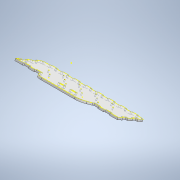
# Autodesk Inventor part: wooden_top
Saved by Autodesk Inventor 2020 (Build 240168000, 168)
## iProperties
Created: 2019-07-24
Part Number: wooden_top
Material: Generic
Document SubType Name: Modeling
Designer: erwin
Density: 1 g/cm^3
Appearance: Default
Author: erwin
Autodesk Inventor part; units mm, degrees
ref_plane "YZ Plane" through (0, 0, 0) normal (1, 0, 0) x (0, 1, 0)
ref_plane "XZ Plane" through (0, 0, 0) normal (0, 1, 0) x (-1, 0, 0)
ref_plane "XY Plane" through (0, 0, 0) normal (0, 0, 1) x (1, 0, 0)
ref_plane "Work Plane2" through (0, 481.1893, 141.342) normal (0, -0.866, 0.5) x (1, 0, 0)
sketch "Sketch2" plane through (0, 481.1893, 141.342) normal (0, -0.866, 0.5) x (1, 0, 0)
  line L0 (0, 0) -> (0, 36) projected
  line L1 (0, 0) -> (12, 0) projected
  line L2 (12, 36) -> (12, 0) projected
  line L3 (0, 36) -> (12, 36) projected
  line L4 (0, -72) -> (0, -36) projected
  line L5 (0, -72) -> (12, -72) projected
  line L6 (12, -36) -> (12, -72) projected
  line L7 (0, -36) -> (12, -36) projected
  line L8 (0, -144) -> (0, -108) projected
  line L9 (0, -144) -> (12, -144) projected
  line L10 (12, -108) -> (12, -144) projected
  line L11 (0, -108) -> (12, -108) projected
  line L12 (48, -147.6081) -> (12, -147.6081) projected
  line L13 (12, 36) -> (624, 36)
  line L14 (624, 36) -> (624, -164)
  line L15 (624, -164) -> (12, -164)
  line L16 (12, -164) -> (12, 36)
  line L17 (318, -164) -> (318, 36) construction
  line L18 (636, 0) -> (636, 36)
  line L19 (636, 0) -> (624, 0)
  line L20 (624, 36) -> (624, 0)
  line L21 (636, 36) -> (624, 36)
  line L22 (636, -72) -> (636, -36)
  line L23 (636, -72) -> (624, -72)
  line L24 (624, -36) -> (624, -72)
  line L25 (636, -36) -> (624, -36)
  line L26 (636, -144) -> (636, -108)
  line L27 (636, -144) -> (624, -144)
  line L28 (624, -108) -> (624, -144)
  line L29 (636, -108) -> (624, -108)
  line L30 (588, -147.6081) -> (624, -147.6081)
  line L31 (624, -164) -> (624, 36)
  line L32 (12, 36) -> (48, 36)
  line L33 (48, 36) -> (48, 24)
  line L34 (48, 24) -> (12, 24)
  line L35 (12, 24) -> (12, 36)
  line L36 (84, 24) -> (48, 24)
  line L37 (84, 36) -> (84, 24)
  line L38 (48, 36) -> (84, 36)
  line L39 (48, 24) -> (48, 36)
  line L40 (120, 24) -> (84, 24)
  line L41 (120, 36) -> (120, 24)
  line L42 (84, 36) -> (120, 36)
  line L43 (84, 24) -> (84, 36)
  line L44 (156, 24) -> (120, 24)
  line L45 (156, 36) -> (156, 24)
  line L46 (120, 36) -> (156, 36)
  line L47 (120, 24) -> (120, 36)
  line L48 (192, 24) -> (156, 24)
  line L49 (192, 36) -> (192, 24)
  line L50 (156, 36) -> (192, 36)
  line L51 (156, 24) -> (156, 36)
  line L52 (228, 24) -> (192, 24)
  line L53 (228, 36) -> (228, 24)
  line L54 (192, 36) -> (228, 36)
  line L55 (192, 24) -> (192, 36)
  line L56 (264, 24) -> (228, 24)
  line L57 (264, 36) -> (264, 24)
  line L58 (228, 36) -> (264, 36)
  line L59 (228, 24) -> (228, 36)
  line L60 (300, 24) -> (264, 24)
  line L61 (300, 36) -> (300, 24)
  line L62 (264, 36) -> (300, 36)
  line L63 (264, 24) -> (264, 36)
  line L64 (336, 24) -> (300, 24)
  line L65 (336, 36) -> (336, 24)
  line L66 (300, 36) -> (336, 36)
  line L67 (300, 24) -> (300, 36)
  line L68 (372, 24) -> (336, 24)
  line L69 (372, 36) -> (372, 24)
  line L70 (336, 36) -> (372, 36)
  line L71 (336, 24) -> (336, 36)
  line L72 (408, 24) -> (372, 24)
  line L73 (408, 36) -> (408, 24)
  line L74 (372, 36) -> (408, 36)
  line L75 (372, 24) -> (372, 36)
  line L76 (444, 24) -> (408, 24)
  line L77 (444, 36) -> (444, 24)
  line L78 (408, 36) -> (444, 36)
  line L79 (408, 24) -> (408, 36)
  line L80 (480, 24) -> (444, 24)
  line L81 (480, 36) -> (480, 24)
  line L82 (444, 36) -> (480, 36)
  line L83 (444, 24) -> (444, 36)
  line L84 (516, 24) -> (480, 24)
  line L85 (516, 36) -> (516, 24)
  line L86 (480, 36) -> (516, 36)
  line L87 (480, 24) -> (480, 36)
  line L88 (552, 24) -> (516, 24)
  line L89 (552, 36) -> (552, 24)
  line L90 (516, 36) -> (552, 36)
  line L91 (516, 24) -> (516, 36)
  line L92 (588, 24) -> (552, 24)
  line L93 (588, 36) -> (588, 24)
  line L94 (552, 36) -> (588, 36)
  line L95 (552, 24) -> (552, 36)
  line L96 (624, 24) -> (588, 24)
  line L97 (624, 36) -> (624, 24)
  line L98 (588, 36) -> (624, 36)
  line L99 (588, 24) -> (588, 36)
  line L100 (660, 24) -> (624, 24)
  line L101 (660, 36) -> (660, 24)
  line L102 (624, 36) -> (660, 36)
  line L103 (624, 24) -> (624, 36)
  line L104 (696, 24) -> (660, 24)
  line L105 (696, 36) -> (696, 24)
  line L106 (660, 36) -> (696, 36)
  line L107 (660, 24) -> (660, 36)
  line L108 (732, 24) -> (696, 24)
  line L109 (732, 36) -> (732, 24)
  line L110 (696, 36) -> (732, 36)
  line L111 (696, 24) -> (696, 36)
  line L112 (12, -64) -> (624, -64) construction
  line L113 (12, -164) -> (12, -128)
  line L114 (12, -164) -> (624, -164)
  line L115 (12, -164) -> (48, -164)
  line L116 (48, -164) -> (48, -152)
  line L117 (48, -152) -> (12, -152)
  line L118 (12, -152) -> (12, -164)
  line L119 (84, -152) -> (48, -152)
  line L120 (84, -164) -> (84, -152)
  line L121 (48, -164) -> (84, -164)
  line L122 (48, -152) -> (48, -164)
  line L123 (120, -152) -> (84, -152)
  line L124 (120, -164) -> (120, -152)
  line L125 (84, -164) -> (120, -164)
  line L126 (84, -152) -> (84, -164)
  line L127 (156, -152) -> (120, -152)
  line L128 (156, -164) -> (156, -152)
  line L129 (120, -164) -> (156, -164)
  line L130 (120, -152) -> (120, -164)
  line L131 (192, -152) -> (156, -152)
  line L132 (192, -164) -> (192, -152)
  line L133 (156, -164) -> (192, -164)
  line L134 (156, -152) -> (156, -164)
  line L135 (228, -152) -> (192, -152)
  line L136 (228, -164) -> (228, -152)
  line L137 (192, -164) -> (228, -164)
  line L138 (192, -152) -> (192, -164)
  line L139 (264, -152) -> (228, -152)
  line L140 (264, -164) -> (264, -152)
  line L141 (228, -164) -> (264, -164)
  line L142 (228, -152) -> (228, -164)
  line L143 (300, -152) -> (264, -152)
  line L144 (300, -164) -> (300, -152)
  line L145 (264, -164) -> (300, -164)
  line L146 (264, -152) -> (264, -164)
  line L147 (336, -152) -> (300, -152)
  line L148 (336, -164) -> (336, -152)
  line L149 (300, -164) -> (336, -164)
  line L150 (300, -152) -> (300, -164)
  line L151 (372, -152) -> (336, -152)
  line L152 (372, -164) -> (372, -152)
  line L153 (336, -164) -> (372, -164)
  line L154 (336, -152) -> (336, -164)
  line L155 (408, -152) -> (372, -152)
  line L156 (408, -164) -> (408, -152)
  line L157 (372, -164) -> (408, -164)
  line L158 (372, -152) -> (372, -164)
  line L159 (444, -152) -> (408, -152)
  line L160 (444, -164) -> (444, -152)
  line L161 (408, -164) -> (444, -164)
  line L162 (408, -152) -> (408, -164)
  line L163 (480, -152) -> (444, -152)
  line L164 (480, -164) -> (480, -152)
  line L165 (444, -164) -> (480, -164)
  line L166 (444, -152) -> (444, -164)
  line L167 (516, -152) -> (480, -152)
  line L168 (516, -164) -> (516, -152)
  line L169 (480, -164) -> (516, -164)
  line L170 (480, -152) -> (480, -164)
  line L171 (552, -152) -> (516, -152)
  line L172 (552, -164) -> (552, -152)
  line L173 (516, -164) -> (552, -164)
  line L174 (516, -152) -> (516, -164)
  line L175 (588, -152) -> (552, -152)
  line L176 (588, -164) -> (588, -152)
  line L177 (552, -164) -> (588, -164)
  line L178 (552, -152) -> (552, -164)
  line L179 (624, -152) -> (588, -152)
  line L180 (624, -164) -> (624, -152)
  line L181 (588, -164) -> (624, -164)
  line L182 (588, -152) -> (588, -164)
  line L183 (624, -152) -> (624, -164)
  circle A0 centre (318, -64) radius 2.5
  circle A1 centre (218, -64) radius 2.5
  circle A2 centre (118, -64) radius 2.5
  line L184 (624, -64) -> (12, -64) construction
  circle A3 centre (318, -64) radius 2.5
  circle A4 centre (418, -64) radius 2.5
  circle A5 centre (518, -64) radius 2.5
  circle A6 centre (168, -14) radius 2.5
  circle A7 centre (268, -14) radius 2.5
  circle A8 centre (468, -14) radius 2.5
  circle A9 centre (368, -14) radius 2.5
  line L185 (318, 36) -> (318, -164) construction
  circle A10 centre (168, -114) radius 2.5
  circle A11 centre (268, -114) radius 2.5
  circle A12 centre (468, -114) radius 2.5
  circle A13 centre (368, -114) radius 2.5
  point P0 (0, -363.0004)
  point P1 (48, 24)
  point P2 (12, 0)
  point P3 (12, -72)
  point P4 (12, -108)
  point P5 (12, -144)
  point P6 (12, -152)
  point P7 (48, -164)
  point P8 (84, -164)
  point P9 (84, -152)
  point P10 (120, -164)
  point P11 (156, -164)
  point P12 (156, -152)
  point P13 (192, -164)
  point P14 (228, -164)
  point P15 (228, -152)
  point P16 (264, -164)
  point P17 (300, -164)
  point P18 (300, -152)
  point P19 (336, -164)
  point P20 (372, -164)
  point P21 (372, -152)
  point P22 (408, -164)
  point P23 (444, -164)
  point P24 (444, -152)
  point P25 (480, -164)
  point P26 (516, -164)
  point P27 (516, -152)
  point P28 (552, -164)
  point P29 (588, -164)
  point P30 (624, -144)
  point P31 (624, -108)
  point P32 (624, -72)
  point P33 (624, -36)
  point P34 (624, 0)
  point P35 (552, 24)
  point P36 (552, 36)
  point P37 (516, 36)
  point P38 (480, 24)
  point P39 (480, 36)
  point P40 (444, 36)
  point P41 (408, 36)
  point P42 (372, 36)
  point P43 (336, 24)
  point P44 (336, 36)
  point P45 (300, 36)
  point P46 (264, 24)
  point P47 (264, 36)
  point P48 (228, 36)
  point P49 (192, 24)
  point P50 (192, 36)
  point P51 (156, 36)
  point P52 (120, 24)
  point P53 (120, 36)
  point P54 (84, 36)
  dimension "d4" = 612
  dimension "d5" = 200
  dimension "d6" = 12
  dimension "d7" = 36
  dimension "d10" = 36
  dimension "d21" = 5
  dimension "d24" = 100
  dimension "d29" = 5
  dimension "d30" = 5
  dimension "d31" = 100
  dimension "d32" = 50
  dimension "d33" = 50
  constraints: 346 end point, 96 symmetric about line, 14 centre point, 5 midpoint, 4 horizontal, 4 parallel, 2 perpendicular, 1 collinear, 164 other
  measures "d4" distance of L14.end L15.end
  measures "d5" distance of L13.end L14.end
  measures "d6" distance of L32.end L33.end
  measures "d7" distance of L33.end L34.end
  measures "d10" distance of L34.end L36.end
  measures "d21" diameter of A0
  measures "d24" distance of A0.centre A1.centre
  measures "d29" diameter of A6
  measures "d30" diameter of A7
  measures "d31" distance of A6.centre A7.centre
  measures "d32" distance from line of L17 A7.centre
  measures "d33" horizontal distance of A0.centre A7.centre
extrude "Extrusion2" add sketch "Sketch2" along normal blind 12 contours L0 L3 L2 L1 | L2 L34 L36 L40 L44 L48 L52 L56 L60 L64 L68 L72 L76 L80 L84 L88 L92 L96 L14 L179 L175 L171 L167 L163 L159 L155 L151 L147 L143 L139 L135 L131 L127 L123 L119 L117 L16 L10 L6 | L13 L33 L34 L2 | L6 L5 L4 L7 | L13 L41 L40 L37 | L10 L9 L8 L11 | L13 L49 L48 L45 | L13 L53 L52 L49 | L13 L57 L56 L53 | L119 L120 L15 L116 | L13 L65 L64 L61 | L127 L128 L15 L124 | L13 L73 L72 L69 | L13 L77 L76 L73 | L135 L136 L15 L132 | L13 L81 L80 L77 | L143 L144 L15 L140 | L13 L89 L88 L85 | L151 L152 L15 L148 | L13 L14 L96 L93 | L21 L18 L100 L14 | L100 L18 L19 L14 | L159 L160 L15 L156 | L25 L22 L23 L14 | L167 L168 L15 L164 | L29 L26 L27 L14 | L175 L176 L15 L172
sketch "Sketch3" plane through (0, 470.797, 147.342) normal (0, -0.866, 0.5) x (1, 0, 0)
  line L0 (588, -164) -> (588, -152) projected
  line L1 (588, -152) -> (624, -152) projected
  line L2 (624, -152) -> (624, -144) projected
  line L3 (624, -144) -> (636, -144) projected
  line L4 (636, -144) -> (636, -108) projected
  line L5 (636, -108) -> (624, -108) projected
  line L6 (624, -108) -> (624, -72) projected
  line L7 (624, -72) -> (636, -72) projected
  line L8 (636, -72) -> (636, -36) projected
  line L9 (636, -36) -> (624, -36) projected
  line L10 (624, -36) -> (624, 0) projected
  line L11 (624, 0) -> (636, 0) projected
  line L12 (636, 0) -> (636, 36) projected
  line L13 (636, 36) -> (588, 36) projected
  line L14 (588, 36) -> (588, 24) projected
  line L15 (588, 24) -> (552, 24) projected
  line L16 (552, 24) -> (552, 36) projected
  line L17 (552, 36) -> (516, 36) projected
  line L18 (516, 36) -> (516, 24) projected
  line L19 (516, 24) -> (480, 24) projected
  line L20 (480, 24) -> (480, 36) projected
  line L21 (264, 36) -> (156, 36) projected
  line L22 (480, 36) -> (372, 36) projected
  line L23 (372, 36) -> (372, 24) projected
  line L24 (372, 24) -> (336, 24) projected
  line L25 (336, 24) -> (336, 36) projected
  line L26 (336, 36) -> (300, 36) projected
  line L27 (300, 36) -> (300, 24) projected
  line L28 (300, 24) -> (264, 24) projected
  line L29 (264, 24) -> (264, 36) projected
  line L30 (156, 36) -> (156, 24) projected
  line L31 (156, 24) -> (120, 24) projected
  line L32 (120, 24) -> (120, 36) projected
  line L33 (120, 36) -> (84, 36) projected
  line L34 (84, 36) -> (84, 24) projected
  line L35 (84, 24) -> (48, 24) projected
  line L36 (48, 24) -> (48, 36) projected
  line L37 (48, 36) -> (0, 36) projected
  line L38 (0, 36) -> (0, 0) projected
  line L39 (0, 0) -> (12, 0) projected
  line L40 (12, 0) -> (12, -36) projected
  line L41 (12, -36) -> (0, -36) projected
  line L42 (0, -36) -> (0, -72) projected
  line L43 (0, -72) -> (12, -72) projected
  line L44 (12, -72) -> (12, -108) projected
  line L45 (12, -108) -> (0, -108) projected
  line L46 (0, -108) -> (0, -144) projected
  line L47 (0, -144) -> (12, -144) projected
  line L48 (12, -144) -> (12, -152) projected
  line L49 (12, -152) -> (48, -152) projected
  line L50 (48, -152) -> (48, -164) projected
  line L51 (48, -164) -> (84, -164) projected
  line L52 (84, -164) -> (84, -152) projected
  line L53 (84, -152) -> (120, -152) projected
  line L54 (120, -152) -> (120, -164) projected
  line L55 (120, -164) -> (156, -164) projected
  line L56 (156, -164) -> (156, -152) projected
  line L57 (156, -152) -> (192, -152) projected
  line L58 (192, -152) -> (192, -164) projected
  line L59 (192, -164) -> (228, -164) projected
  line L60 (228, -164) -> (228, -152) projected
  line L61 (228, -152) -> (264, -152) projected
  line L62 (264, -152) -> (264, -164) projected
  line L63 (264, -164) -> (300, -164) projected
  line L64 (300, -164) -> (300, -152) projected
  line L65 (300, -152) -> (336, -152) projected
  line L66 (336, -152) -> (336, -164) projected
  line L67 (336, -164) -> (372, -164) projected
  line L68 (372, -164) -> (372, -152) projected
  line L69 (372, -152) -> (408, -152) projected
  line L70 (408, -152) -> (408, -164) projected
  line L71 (408, -164) -> (444, -164) projected
  line L72 (444, -164) -> (444, -152) projected
  line L73 (444, -152) -> (480, -152) projected
  line L74 (480, -152) -> (480, -164) projected
  line L75 (480, -164) -> (516, -164) projected
  line L76 (516, -164) -> (516, -152) projected
  line L77 (516, -152) -> (552, -152) projected
  line L78 (552, -152) -> (552, -164) projected
  line L79 (552, -164) -> (588, -164) projected
  line L80 (156, 36) -> (167.3747, 64.5218)
  line L81 (213.8176, 96) -> (422.1824, 96)
  line L82 (468.6253, 64.5218) -> (480, 36)
  arc A0 (213.8176, 96) -> (167.3747, 64.5218) centre (213.8176, 46) ccw
  arc A1 (468.6253, 64.5218) -> (422.1824, 96) centre (422.1824, 46) ccw
  line L83 (336, 36) -> (300, 36) projected
  line L84 (156, 36) -> (480, 36)
  point P0 (0, -363.0004)
  point P1 (300, 36)
  dimension "d17" = 50
  dimension "d20" = 60
  constraints: 8 end point, 4 point on circle, 4 tangent, 2 centre point, 1 collinear, 1 equal length, 1 equal radius, 1 horizontal, 1 parallel
  measures "d17" radius of A0
  measures "d20" distance between parallel lines of L26 L81
extrude "Extrusion3" add sketch "Sketch3" against normal blind 12 contours L22 L84 L26 L21 L80 A0 L81 A1 L82
sketch "Sketch5" plane through (0, 481.1893, 141.342) normal (0, 0.866, -0.5) x (1, 0, 0)
  line L0 (264, -24) -> (264, -36) projected
  line L1 (300, -24) -> (264, -24) projected
  line L2 (300, -36) -> (300, -24) projected
  line L3 (300, -36) -> (264, -36) projected
  line L4 (336, -24) -> (336, -36) projected
  line L5 (372, -24) -> (336, -24) projected
  line L6 (372, -36) -> (372, -24) projected
  line L7 (372, -36) -> (336, -36) projected
  line L8 (156, -36) -> (167.3747, -64.5218) projected
  arc A0 (167.3747, -64.5218) -> (213.8176, -96) centre (213.8176, -46) ccw projected
  line L9 (213.8176, -96) -> (422.1824, -96) projected
  arc A1 (422.1824, -96) -> (468.6253, -64.5218) centre (422.1824, -46) ccw projected
  line L10 (468.6253, -64.5218) -> (480, -36) projected
  line L11 (480, -24) -> (480, -36) projected
  line L12 (516, -24) -> (480, -24) projected
  line L13 (516, -36) -> (516, -24) projected
  line L14 (552, -36) -> (516, -36) projected
  line L15 (552, -24) -> (552, -36) projected
  line L16 (588, -24) -> (552, -24) projected
  line L17 (588, -36) -> (588, -24) projected
  line L18 (636, -36) -> (588, -36) projected
  line L19 (636, 0) -> (636, -36) projected
  line L20 (624, 0) -> (636, 0) projected
  line L21 (624, 36) -> (624, 0) projected
  line L22 (636, 36) -> (624, 36) projected
  line L23 (636, 72) -> (636, 36) projected
  line L24 (624, 72) -> (636, 72) projected
  line L25 (624, 108) -> (624, 72) projected
  line L26 (636, 108) -> (624, 108) projected
  line L27 (636, 144) -> (636, 108) projected
  line L28 (624, 144) -> (636, 144) projected
  line L29 (624, 152) -> (624, 144) projected
  line L30 (588, 152) -> (624, 152) projected
  line L31 (588, 164) -> (588, 152) projected
  line L32 (552, 164) -> (588, 164) projected
  line L33 (552, 152) -> (552, 164) projected
  line L34 (516, 152) -> (552, 152) projected
  line L35 (516, 164) -> (516, 152) projected
  line L36 (480, 164) -> (516, 164) projected
  line L37 (480, 152) -> (480, 164) projected
  line L38 (444, 152) -> (480, 152) projected
  line L39 (444, 164) -> (444, 152) projected
  line L40 (408, 164) -> (444, 164) projected
  line L41 (408, 152) -> (408, 164) projected
  line L42 (372, 152) -> (408, 152) projected
  line L43 (372, 164) -> (372, 152) projected
  line L44 (336, 164) -> (372, 164) projected
  line L45 (336, 152) -> (336, 164) projected
  line L46 (300, 152) -> (336, 152) projected
  line L47 (300, 164) -> (300, 152) projected
  line L48 (264, 164) -> (300, 164) projected
  line L49 (264, 152) -> (264, 164) projected
  line L50 (228, 152) -> (264, 152) projected
  line L51 (228, 164) -> (228, 152) projected
  line L52 (192, 164) -> (228, 164) projected
  line L53 (192, 152) -> (192, 164) projected
  line L54 (156, 152) -> (192, 152) projected
  line L55 (156, 164) -> (156, 152) projected
  line L56 (120, 164) -> (156, 164) projected
  line L57 (120, 152) -> (120, 164) projected
  line L58 (84, 152) -> (120, 152) projected
  line L59 (84, 164) -> (84, 152) projected
  line L60 (48, 164) -> (84, 164) projected
  line L61 (48, 152) -> (48, 164) projected
  line L62 (12, 152) -> (48, 152) projected
  line L63 (12, 144) -> (12, 152) projected
  line L64 (0, 144) -> (12, 144) projected
  line L65 (0, 108) -> (0, 144) projected
  line L66 (12, 108) -> (0, 108) projected
  line L67 (12, 72) -> (12, 108) projected
  line L68 (0, 72) -> (12, 72) projected
  line L69 (0, 36) -> (0, 72) projected
  line L70 (12, 36) -> (0, 36) projected
  line L71 (12, 0) -> (12, 36) projected
  line L72 (0, 0) -> (12, 0) projected
  line L73 (0, -36) -> (0, 0) projected
  line L74 (48, -36) -> (0, -36) projected
  line L75 (48, -24) -> (48, -36) projected
  line L76 (84, -24) -> (48, -24) projected
  line L77 (84, -36) -> (84, -24) projected
  line L78 (120, -36) -> (84, -36) projected
  line L79 (120, -24) -> (120, -36) projected
  line L80 (156, -24) -> (120, -24) projected
  line L81 (156, -36) -> (156, -24) projected
  circle A2 centre (368, 114) radius 2.5 projected
  circle A3 centre (168, 114) radius 2.5 projected
  circle A4 centre (468, 14) radius 2.5 projected
  circle A5 centre (268, 14) radius 2.5 projected
  circle A6 centre (168, 14) radius 2.5 projected
  circle A7 centre (418, 64) radius 2.5 projected
  circle A8 centre (518, 64) radius 2.5 projected
  circle A9 centre (118, 64) radius 2.5 projected
  circle A10 centre (218, 64) radius 2.5 projected
  circle A11 centre (318, 64) radius 2.5 projected
  circle A12 centre (368, 14) radius 2.5 projected
  circle A13 centre (268, 114) radius 2.5 projected
  circle A14 centre (468, 114) radius 2.5 projected
  point P0 (0, 363.0004)
equation "\"d4\" = 17 * d7"
equation "\"d7\" = 3 * d6"
equation "\"d10\" = d7"
equation "\"d31\" = d24"
equation "\"d32\" = 0.5 * d31"
equation "\"d33\" = d32"
body "Solid1"
